Autodesk Inventor part; units mm, degrees
(part 2 of 2)
sketch "Эскиз22" plane through (0, 0, 3) normal (0, 0, 1) x (1, 0, 0)
  line L0 (-56.7398, -37.5269) -> (-56.7398, -39.6669) projected
  line L1 (-56.7398, -39.6669) -> (-56.5398, -39.8669) projected
  line L2 (-56.5398, -39.8669) -> (-54.3998, -39.8669) projected
  line L3 (-54.3998, -39.8669) -> (-54.1998, -39.6669) projected
  line L4 (-54.1998, -39.6669) -> (-54.1998, -37.5269) projected
  line L5 (-54.1998, -37.5269) -> (-54.3998, -37.3269) projected
  line L6 (-54.3998, -37.3269) -> (-56.5398, -37.3269) projected
  line L7 (-56.5398, -37.3269) -> (-56.7398, -37.5269) projected
  line L8 (-55.1498, -38.9169) -> (-55.1498, -38.2769) projected
  line L9 (-55.7898, -38.9169) -> (-55.1498, -38.9169) projected
  line L10 (-55.7898, -38.2769) -> (-55.7898, -38.9169) projected
  line L11 (-55.1498, -38.2769) -> (-55.7898, -38.2769) projected
  line L12 (-56.7398, -32.4469) -> (-56.7398, -34.5869) projected
  line L13 (-56.7398, -34.5869) -> (-56.5398, -34.7869) projected
  line L14 (-56.5398, -34.7869) -> (-54.3998, -34.7869) projected
  line L15 (-54.3998, -34.7869) -> (-54.1998, -34.5869) projected
  line L16 (-54.1998, -34.5869) -> (-54.1998, -32.4469) projected
  line L17 (-54.1998, -32.4469) -> (-54.3998, -32.2469) projected
  line L18 (-54.3998, -32.2469) -> (-56.5398, -32.2469) projected
  line L19 (-56.5398, -32.2469) -> (-56.7398, -32.4469) projected
  line L20 (-55.1498, -33.8369) -> (-55.1498, -33.1969) projected
  line L21 (-55.7898, -33.8369) -> (-55.1498, -33.8369) projected
  line L22 (-55.7898, -33.1969) -> (-55.7898, -33.8369) projected
  line L23 (-55.1498, -33.1969) -> (-55.7898, -33.1969) projected
  line L24 (-55.4698, -32.2469) -> (-55.4698, -34.7869)
  line L25 (-55.4698, -37.3269) -> (-55.4698, -39.8669)
  circle A0 centre (-55.4698, -38.5969) radius 2.5
  circle A1 centre (-55.4698, -33.5169) radius 2.5
  line L26 (-57.9698, -33.5169) -> (-57.9698, -38.5969)
  line L27 (-52.9698, -38.5969) -> (-52.9698, -33.5169)
  point P0 (0, 0)
  dimension "d155" = 5
  dimension "d156" = 5
  constraints: 8 end point, 6 midpoint, 4 point on circle, 2 centre point, 2 tangent
  measures "d155" diameter of A0
  measures "d156" diameter of A1
extrude "Вырез15" cut sketch "Эскиз22" against normal blind 3 contours L7 L6 L25 L11 L10 L9 L2 L1 L0 | L6 L5 L4 L3 L2 L25 L9 L8 L11 | L25 L9 L10 L11 | L11 L8 L9 L25 | L19 L18 L24 L23 L22 L21 L14 L13 L12 | L18 L17 L16 L15 L14 L24 L21 L20 L23 | L24 L21 L22 L23 | L23 L20 L21 L24 | A0 | A0 L26 A1 L27 | A1
sketch "Эскиз23" plane through (0, 0, 3) normal (0, 0, 1) x (1, 0, 0)
  circle A0 centre (-67, -50) radius 1.6 projected
  circle A1 centre (-67, 50) radius 1.6 projected
  circle A2 centre (-67, 50) radius 1.35
  circle A3 centre (-67, -50) radius 1.35
  point P0 (0, 0)
  dimension "d157" = 2.7
  dimension "d158" = 2.7
  constraints: 2 centre point, 2 coincident
  measures "d157" diameter of A2
  measures "d158" diameter of A3
extrude "Вырез16" cut sketch "Эскиз23" against normal blind 3 contours A2 | A3
sketch "Эскиз24" plane through (0, 0, 0) normal (0, 0, -1) x (-1, 0, 0)
  line L0 (79, 26) -> (79, -26) projected
  line L1 (55.8, 26) -> (79, 26) projected
  line L2 (55.8, -26) -> (55.8, 26) projected
  line L3 (79, -26) -> (55.8, -26) projected
  line L4 (76, 23) -> (76, -23)
  line L5 (76, -23) -> (58.8, -23)
  line L6 (58.8, -23) -> (58.8, 23)
  line L7 (58.8, 23) -> (76, 23)
  line L8 (73.9, 23) -> (60.9, 23)
  line L9 (60.9, 23) -> (60.9, -23)
  line L10 (60.9, -23) -> (73.9, -23)
  line L11 (73.9, -23) -> (73.9, 23)
  line L12 (67.4, 26) -> (67.4, 23)
  line L13 (60.9, -23) -> (73.9, -23)
  line L14 (73.9, -23) -> (73.9, -29)
  line L15 (73.9, -29) -> (60.9, -29)
  line L16 (60.9, -29) -> (60.9, -23)
  line L17 (73.9, 23) -> (60.9, 23)
  line L18 (60.9, 23) -> (60.9, -29)
  line L19 (60.9, -29) -> (73.9, -29)
  line L20 (73.9, -29) -> (73.9, 23)
  line L21 (60.9, 23) -> (73.9, 23)
  line L22 (73.9, 23) -> (73.9, 29)
  line L23 (73.9, 29) -> (60.9, 29)
  line L24 (60.9, 29) -> (60.9, 23)
  ellipse E0 centre (45.8314, 13.2) end of major axis (31.7971, 13.2) minor radius 4.8 (59.8656, 13.2) -> (59.7, 13.9353) ccw projected
  line L25 (59.8656, -1.3) -> (59.8656, 13.2) projected
  ellipse E1 centre (45.8314, -1.3) end of major axis (59.8656, -1.3) minor radius 4.8 (59.7, -2.0353) -> (59.8656, -1.3) ccw projected
  line L26 (59.7, -28.1138) -> (59.7, -2.0353) projected
  line L27 (74, -28.1138) -> (59.7, -28.1138) projected
  line L28 (74, 28.1138) -> (74, -28.1138) projected
  line L29 (59.7, 28.1138) -> (74, 28.1138) projected
  line L30 (59.7, 13.9353) -> (59.7, 28.1138) projected
  point P0 (0, 0)
  dimension "d161" = 3
  dimension "d162" = 13
  dimension "d163" = 3
  dimension "d174" = 3
  constraints: 42 end point, 8 parallel, 5 perpendicular, 4 horizontal, 2 collinear, 2 midpoint, 2 point on line, 5 other
  measures "d161" distance between parallel lines of L1 L7
  measures "d162" distance between parallel lines of L9 L11
  measures "d163" distance between parallel lines of L15 L3
  measures "d174" distance between parallel lines of L1 L23
extrude "Вырез17" cut sketch "Эскиз24" against normal blind 3 contours L22 L7 L12 L1 | L1 L24 L29 L22 | L14 L27 L16 L3 | L3 L16 L5 L14 | L12 L7 L24 L1 | L11 L5 L9 L7 | L29 L24 L23 L22 | L14 L15 L16 L27
fillet "Сопряжение7" radius 3 4 edges at (-60.9, -29, 1.5) (-73.9, 29, 1.5) (-60.9, 29, 1.5) (-73.9, -29, 1.5)
sketch "Эскиз27" plane through (0, 0, 0) normal (0, 0, -1) x (-1, 0, 0)
  circle A0 centre (35.6204, 24.4819) radius 1.6 projected
  circle A1 centre (35.6204, -18.5319) radius 1.6 projected
  line L0 (37.9733, 32.408) -> (23.7204, 32.408) projected
  line L1 (23.7204, 32.408) -> (23.7204, 28.408) projected
  line L2 (23.7204, 28.408) -> (23.0463, 28.408) projected
  line L3 (23.0463, 28.408) -> (23.0463, 10.238) projected
  ellipse E0 centre (48.7746, 0) end of major axis (9.3032, 0) minor radius 13.5 (27.0101, 11.2623) -> (23.0463, 10.238) ccw projected
  line L4 (27.0101, 11.2623) -> (27.0101, -11.2623) projected
  ellipse E1 centre (48.7746, 0) end of major axis (9.3032, 0) minor radius 13.5 (23.0463, -10.238) -> (27.0101, -11.2623) ccw projected
  line L5 (23.0463, -10.238) -> (23.0463, -28.408) projected
  line L6 (23.0463, -28.408) -> (23.7204, -28.408) projected
  line L7 (23.7204, -28.408) -> (23.7204, -29.6) projected
  line L8 (23.7204, -29.6) -> (37.667, -29.6) projected
  line L9 (37.667, -29.6) -> (37.667, -40.6) projected
  line L10 (37.667, -40.6) -> (23.7204, -40.6) projected
  line L11 (23.7204, -40.6) -> (23.7204, -43.5) projected
  line L12 (23.7204, -43.5) -> (38.2118, -43.5) projected
  line L13 (38.2118, -43.5) -> (38.1494, -40.6) projected
  line L14 (38.1494, -40.6) -> (37.9129, -40.6) projected
  line L15 (37.9129, -29.6) -> (37.9129, -40.6) projected
  line L16 (37.9129, -29.6) -> (37.8873, -28.408) projected
  line L17 (37.8873, -28.408) -> (39.6204, -28.408) projected
  line L18 (39.6204, -28.408) -> (39.6204, -5.9502) projected
  ellipse E2 centre (47.0551, -1.3) end of major axis (31.559, -1.3) minor radius 5.3 (31.559, -1.3) -> (39.6204, -5.9502) ccw projected
  line L19 (31.559, 13.2) -> (31.559, -1.3) projected
  ellipse E3 centre (47.0551, 13.2) end of major axis (31.559, 13.2) minor radius 5.3 (39.6204, 17.8502) -> (31.559, 13.2) ccw projected
  line L20 (39.6204, 17.8502) -> (39.6204, 28.408) projected
  line L21 (39.6204, 28.408) -> (37.8873, 28.408) projected
  line L22 (37.9733, 32.408) -> (37.8873, 28.408) projected
  circle A2 centre (35.6204, -18.5319) radius 1.5
  circle A3 centre (35.6204, 24.4819) radius 1.5
  point P0 (0, 0)
  dimension "d175" = 3
  dimension "d176" = 3
  constraints: 2 centre point, 2 coincident, 4 other
  measures "d175" diameter of A2
  measures "d176" diameter of A3
extrude "Вырез19" cut sketch "Эскиз27" against normal blind 3 contours A2 | A3
sketch "Эскиз28" plane through (0, 0, 0) normal (0, 0, -1) x (-1, 0, 0)
  circle A0 centre (-50.4725, -40) radius 2.1 projected
  circle A1 centre (-50.4725, 40) radius 2.1 projected
  circle A2 centre (-50.4725, -40) radius 1.5
  circle A3 centre (-50.4725, 40) radius 1.5
  point P0 (0, 0)
  dimension "d179" = 3
  dimension "d180" = 3
  constraints: 2 centre point, 2 coincident
  measures "d179" diameter of A2
  measures "d180" diameter of A3
extrude "Вырез20" cut sketch "Эскиз28" against normal blind 3 contours A2 | A3
equation "\"d30\" = Толщина"
equation "\"d38\" = Толщина"
equation "\"d58\" = Толщина"
equation "\"d62\" = Толщина"
equation "\"d74\" = Толщина"
equation "\"d82\" = Толщина"
equation "\"d94\" = Толщина"
equation "\"d118\" = Толщина"
equation "\"d11\" = Толщина"
equation "\"d25\" = Радиус_гибки"
equation "\"d26\" = Ширина_просечки"
equation "\"d28\" = Мин_остаток"
equation "\"d27\" = Глубина_просечки"
equation "\"d29\" = Радиус_перехода"
equation "\"d40\" = Радиус_гибки"
equation "\"d41\" = Ширина_просечки"
equation "\"d43\" = Мин_остаток"
equation "\"d42\" = Глубина_просечки"
equation "\"d44\" = Радиус_перехода"
equation "\"d47\" = Радиус_гибки"
equation "\"d48\" = Ширина_просечки"
equation "\"d50\" = Мин_остаток"
equation "\"d49\" = Глубина_просечки"
equation "\"d51\" = Радиус_перехода"
equation "\"d64\" = Радиус_гибки"
equation "\"d65\" = Ширина_просечки"
equation "\"d67\" = Мин_остаток"
equation "\"d66\" = Глубина_просечки"
equation "\"d68\" = Радиус_перехода"
equation "\"Радиус_гибки\" = Толщина"
equation "\"Ширина_просечки\" = Толщина"
equation "\"Глубина_просечки\" = 0.5 * Толщина"
equation "\"Размер_просечки\" = 4 * Толщина"
equation "\"Мин_остаток\" = 2 * Толщина"
equation "\"Радиус_перехода\" = Радиус_гибки"
equation "\"Радиус_Якоби\" = Радиус_гибки"
equation "\"Размер_зазора\" = Толщина"
equation "\"Толщина\" = 3"
